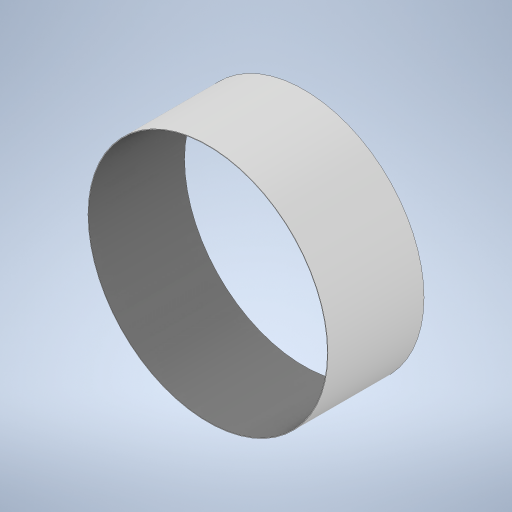
# Autodesk Inventor part: Polycarbonate Track
Saved by Autodesk Inventor 2024 (Build 280153000, 153)
## iProperties
Created: 2021-11-12
Part Number: Polycarbonate Track
Material: PVC, Unplasticized
Document SubType Name: Modeling
Designer: gnzak
Density: 1.29 g/cm^3
Appearance: Default
Author: gnzak
Autodesk Inventor part; units mm, degrees
ref_plane "YZ Plane" through (0, 0, 0) normal (1, 0, 0) x (0, 1, 0)
ref_plane "XZ Plane" through (0, 0, 0) normal (0, 1, 0) x (-1, 0, 0)
sketch "Sketch1" plane through (0, 0, 0) normal (0, 0, 1) x (1, 0, 0)
  circle A0 centre (0, 0) radius 94.742
  circle A1 centre (0, 0) radius 95.25
  dimension "d0" = 0.508
  dimension "d1" = 190.5
  constraints: 2 centre point, 2 coincident
  measures "d0" radial gap between concentric circles of A1 A0
  measures "d1" diameter of A1
extrude "Extrusion1" add sketch "Sketch1" along normal blind 76.2
ref_plane "Work Plane1" through (0, 0, 38.1) normal (0, 0, 1) x (1, 0, 0)
body "Solid1"
